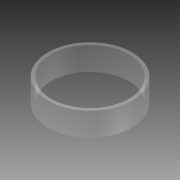
# Autodesk Inventor part: OpenROV 2_3 Dev Duct
Saved by Autodesk Inventor 2012 (Build 160160000, 160)
## iProperties
Created: 2012-03-16
Part Number: OpenROV 2_3 Dev Duct
Material: Polycarbonate, Clear
Document SubType Name: Modeling
Designer: user
Mass: 21.8518 g
Surface Area: 130.542 cm^2
Volume: 18.2098 cm^3
Density: 1.2 g/cm^3
Author: user
Autodesk Inventor part; units mm, degrees
ref_plane "YZ Plane" through (0, 0, 0) normal (1, 0, 0) x (0, 1, 0)
ref_plane "XZ Plane" through (0, 0, 0) normal (0, 1, 0) x (-1, 0, 0)
ref_plane "XY Plane" through (0, 0, 0) normal (0, 0, 1) x (1, 0, 0)
sketch "Sketch1" plane through (0, 0, 0) normal (0, 0, 1) x (1, 0, 0)
  circle A0 centre (0, 0) radius 38.1
  circle A1 centre (0, 0) radius 41.275
  dimension "d0" = 76.2
  dimension "d1" = 82.55
  constraints: 2 centre point, 2 coincident
  measures "d0" diameter of A0
  measures "d1" diameter of A1
extrude "Extrusion1" add sketch "Sketch1" along normal blind 23
body "Solid1"
